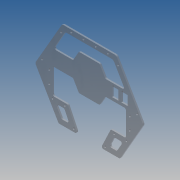
# Autodesk Inventor part: Top Plat
Saved by Autodesk Inventor 2017 (Build 210142000, 142)
## iProperties
Created: 2016-10-14
Part Number: Top Plat
Material: Polycarbonate, Clear
Document SubType Name: Modeling
Designer: James Yelland
Density: 1.2 g/cm^3
Appearance: Polycarbonate - Clear
Author: James Yelland
Autodesk Inventor part; units mm, degrees
ref_plane "YZ Plane" through (0, 0, 0) normal (1, 0, 0) x (0, 1, 0)
ref_plane "XZ Plane" through (0, 0, 0) normal (0, 1, 0) x (-1, 0, 0)
ref_plane "XY Plane" through (0, 0, 0) normal (0, 0, 1) x (1, 0, 0)
sketch "Sketch1" plane through (0, 0, 0) normal (0, 1, 0) x (-1, 0, 0)
  circle A0 centre (-30.6147, -73.9104) radius 1.6
  circle A1 centre (-30.6147, -73.9104) radius 1.6
  line L0 (-103.5566, 2.5) -> (-53.9434, 88.4327)
  line L1 (-49.6132, 90.9327) -> (49.6132, 90.9327)
  line L2 (53.9434, 88.4327) -> (103.5566, 2.5)
  arc A2 (-103.5566, 2.5) -> (-103.5566, -2.5) centre (-99.2265, 0) ccw
  arc A3 (-49.6132, 90.9327) -> (-53.9434, 88.4327) centre (-49.6132, 85.9327) ccw
  arc A4 (53.9434, 88.4327) -> (49.6132, 90.9327) centre (49.6132, 85.9327) ccw
  arc A5 (103.5566, -2.5) -> (103.5566, 2.5) centre (99.2265, 0) ccw
  arc A6 (-43.8396, 80.9325) -> (-48.1698, 78.4325) centre (-43.8396, 75.9325) ccw
  circle A7 centre (-30.6147, -73.9104) radius 1.6
  circle A8 centre (-30.6147, -73.9104) radius 1.6
  arc A9 (48.1698, 78.4325) -> (43.8396, 80.9325) centre (43.8396, 75.9325) ccw
  circle A10 centre (35.5991, 85.9437) radius 1.6
  circle A11 centre (-35.5945, 85.9327) radius 1.6
  circle A12 centre (92.2171, 12.1406) radius 1.6
  circle A13 centre (-92.2171, 12.1406) radius 1.6
  line L3 (-18.2679, -8.3495) -> (18.2679, -8.3495)
  line L4 (-62.8455, -53.0133) -> (-54.5333, -67.4106)
  line L5 (59.1367, 11.2915) -> (33.0718, 11.2915)
  line L6 (59.1367, 11.2915) -> (68.2171, 11.2915)
  line L7 (-62.25, 35.5415) -> (-62.25, 17.0415)
  line L8 (-62.25, 17.0415) -> (-74.75, 17.0415)
  line L9 (-74.75, 17.0415) -> (-74.75, 35.5415)
  line L10 (-74.75, 35.5415) -> (-62.25, 35.5415)
  line L11 (30.4737, 9.7915) -> (20.866, -6.8495)
  line L12 (-30.4737, 9.7915) -> (-20.866, -6.8495)
  arc A14 (33.0718, 11.2915) -> (30.4737, 9.7915) centre (33.0718, 8.2915) ccw
  arc A15 (64.417, 41.2915) -> (67.0151, 45.7915) centre (64.417, 44.2915) ccw
  arc A16 (30.4737, 42.7915) -> (33.0718, 41.2915) centre (33.0718, 44.2915) ccw
  arc A17 (18.2679, -8.3495) -> (20.866, -6.8495) centre (18.2679, -5.3495) ccw
  arc A18 (-20.866, -6.8495) -> (-18.2679, -8.3495) centre (-18.2679, -5.3495) ccw
  arc A19 (-30.4737, 9.7915) -> (-33.0718, 11.2915) centre (-33.0718, 8.2915) ccw
  arc A20 (-33.0718, 41.2915) -> (-30.4737, 42.7915) centre (-33.0718, 44.2915) ccw
  arc A21 (-18.2679, 60.9325) -> (-20.866, 59.4325) centre (-18.2679, 57.9325) ccw
  arc A22 (20.866, 59.4325) -> (18.2679, 60.9325) centre (18.2679, 57.9325) ccw
  arc A23 (-67.0151, 45.7915) -> (-64.417, 41.2915) centre (-64.417, 44.2915) ccw
  line L13 (43.8396, 80.9325) -> (-43.8396, 80.9325)
  line L14 (-48.1698, 78.4325) -> (-67.0151, 45.7915)
  line L15 (-64.417, 41.2915) -> (-33.0718, 41.2915)
  line L16 (-30.4737, 42.7915) -> (-20.866, 59.4325)
  line L17 (-18.2679, 60.9325) -> (18.2679, 60.9325)
  line L18 (20.866, 59.4325) -> (30.4737, 42.7915)
  line L19 (33.0718, 41.2915) -> (64.417, 41.2915)
  line L20 (67.0151, 45.7915) -> (48.1698, 78.4325)
  line L21 (-56.75, 35.5415) -> (-56.75, 17.0415)
  line L22 (-56.75, 17.0415) -> (-44.25, 17.0415)
  line L23 (-44.25, 17.0415) -> (-44.25, 35.5415)
  line L24 (-44.25, 35.5415) -> (-56.75, 35.5415)
  circle A24 centre (-55.4009, 75.9081) radius 1.6
  circle A25 centre (55.3868, 75.9325) radius 1.6
  circle A26 centre (-12, 85.9327) radius 1.6
  circle A27 centre (12, 85.9327) radius 1.6
  circle A28 centre (-78.2171, -22.3594) radius 1.6
  circle A29 centre (-78.2171, 1.6406) radius 1.6
  circle A30 centre (78.2171, -22.3594) radius 1.6
  circle A31 centre (78.2171, 1.6406) radius 1.6
  circle A32 centre (-71.7134, -43.5133) radius 1.6
  circle A33 centre (-47.7134, -43.5133) radius 1.6
  arc A34 (71.2171, 8.2915) -> (68.2171, 11.2915) centre (68.2171, 8.2915) ccw
  line L25 (-33.0718, 11.2915) -> (-68.2171, 11.2915)
  line L26 (-68.2171, -38.5133) -> (-43.8241, -38.5133)
  line L27 (-71.2171, 8.2915) -> (-71.2171, -35.5133)
  arc A35 (-68.2171, 11.2915) -> (-71.2171, 8.2915) centre (-68.2171, 8.2915) ccw
  line L28 (-40.5751, -64.621) -> (-47.4299, -50.2237)
  line L29 (-50.1385, -48.5133) -> (-60.2475, -48.5133)
  arc A36 (-41.1155, -40.2237) -> (-43.8241, -38.5133) centre (-43.8241, -41.5133) ccw
  arc A37 (-47.4299, -50.2237) -> (-50.1385, -48.5133) centre (-50.1385, -51.5133) ccw
  arc A38 (-60.2475, -48.5133) -> (-62.8455, -53.0133) centre (-60.2475, -51.5133) ccw
  arc A39 (-71.2171, -35.5133) -> (-68.2171, -38.5133) centre (-68.2171, -35.5133) ccw
  circle A40 centre (30.6147, -73.9104) radius 1.6
  circle A41 centre (30.6147, -73.9104) radius 1.6
  line L30 (60.303, -77.4174) -> (103.5566, -2.5)
  circle A42 centre (30.6147, -73.9104) radius 1.6
  circle A43 centre (30.6147, -73.9104) radius 1.6
  line L31 (62.8455, -53.0133) -> (54.5294, -67.4174)
  circle A44 centre (47.7134, -43.5133) radius 1.6
  circle A45 centre (71.7134, -43.5133) radius 1.6
  line L32 (68.2171, -38.5133) -> (43.8241, -38.5133)
  line L33 (71.2171, -38.5133) -> (41.9298, -38.5133) construction
  line L34 (71.2171, 8.2915) -> (71.2171, -35.5133)
  line L35 (40.5718, -64.6277) -> (47.4299, -50.2237)
  line L36 (50.1385, -48.5133) -> (60.2475, -48.5133)
  arc A46 (43.8241, -38.5133) -> (41.1155, -40.2237) centre (43.8241, -41.5133) ccw
  arc A47 (50.1385, -48.5133) -> (47.4299, -50.2237) centre (50.1385, -51.5133) ccw
  arc A48 (62.8455, -53.0133) -> (60.2475, -48.5133) centre (60.2475, -51.5133) ccw
  arc A49 (68.2171, -38.5133) -> (71.2171, -35.5133) centre (68.2171, -35.5133) ccw
  line L37 (24.7351, -74.6277) -> (41.1155, -40.2237)
  line L38 (32.3467, -78.9174) -> (57.705, -78.9174)
  line L39 (32.3467, -78.9174) -> (27.4437, -78.9174)
  line L40 (45.0258, -68.9174) -> (43.2805, -68.9174)
  line L41 (45.0258, -68.9174) -> (51.9313, -68.9174)
  arc A50 (24.7351, -74.6277) -> (27.4437, -78.9174) centre (27.4437, -75.9174) ccw
  arc A51 (57.705, -78.9174) -> (60.303, -77.4174) centre (57.705, -75.9174) ccw
  arc A52 (51.9313, -68.9174) -> (54.5294, -67.4174) centre (51.9313, -65.9174) ccw
  arc A53 (40.5718, -64.6277) -> (43.2805, -68.9174) centre (43.2805, -65.9174) ccw
  line L42 (-32.3467, -78.9106) -> (-57.7089, -78.9106)
  line L43 (-45.0278, -68.9106) -> (-51.9352, -68.9106)
  line L44 (-45.0278, -68.9106) -> (-43.2837, -68.9106)
  arc A54 (-43.2837, -68.9106) -> (-40.5751, -64.621) centre (-43.2837, -65.9106) ccw
  arc A55 (-54.5333, -67.4106) -> (-51.9352, -68.9106) centre (-51.9352, -65.9106) ccw
  line L45 (-60.307, -77.4106) -> (-103.5566, -2.5)
  line L46 (-41.1155, -40.2237) -> (-26.1, -71.7609)
  line L47 (-26.1, -71.7609) -> (-24.7383, -74.621)
  line L48 (-27.447, -78.9106) -> (-32.3467, -78.9106)
  arc A56 (-27.447, -78.9106) -> (-24.7383, -74.621) centre (-27.447, -75.9106) ccw
  arc A57 (-60.307, -77.4106) -> (-57.7089, -78.9106) centre (-57.7089, -75.9106) ccw
  point P0 (105, 0)
  point P1 (-105, 0)
  point P2 (-52.5, 90.9327)
  point P3 (52.5, 90.9327)
  point P4 (-46.7264, 80.9325)
  point P5 (46.7264, 80.9325)
  point P6 (-50.7681, -73.9321)
  point P7 (-5, -80.9325)
  point P8 (5, -80.9325)
  point P9 (69.6132, 41.2915)
  point P10 (-69.6132, 41.2915)
  point P11 (0, -8.3495)
  point P12 (0, 90.9327)
  point P13 (-59.7134, -39.5133)
  point P14 (-59.7134, -47.5133)
  point P15 (-70.9879, -38.9104)
  point P16 (-62.905, -52.9104)
  point P17 (-38.1553, -69.7034)
  point P18 (54.8095, -86.9325)
  point P19 (50.7681, -73.9321)
  point P20 (59.7134, -47.5133)
  point P21 (59.7134, -39.5133)
  point P22 (70.9879, -38.9104)
  point P23 (62.905, -52.9104)
  point P24 (38.1553, -69.7034)
  point P25 (24.8278, -74.4329)
  point P26 (22.3467, -78.9174)
  point P27 (53.6633, -68.9174)
  point P28 (-38.5327, -68.9106)
  dimension "d252" = 3.2
  dimension "d254" = 3.2
  dimension "d258" = 3.2
  dimension "d259" = 3.2
  dimension "d263" = 3.2
  dimension "d264" = 3.2
  dimension "d268" = 3.2
  dimension "d269" = 3.2
  dimension "d327" = 3.2
  dimension "d328" = 3.2
  dimension "d336" = 3
  dimension "d339" = 3
  constraints: 98 end point, 69 point on circle, 58 centre point, 26 point on line, 23 tangent, 6 equal radius, 4 coincident, 4 horizontal, 2 midpoint, 1 collinear
  measures "d252" diameter of A26
  measures "d254" diameter of A27
  measures "d258" diameter of A28
  measures "d259" diameter of A29
  measures "d263" diameter of A30
  measures "d264" diameter of A31
  measures "d268" diameter of A32
  measures "d269" diameter of A33
  measures "d327" diameter of A45
  measures "d328" diameter of A44
  measures "d336" radius of A50
  measures "d339" radius of A56
extrude "Extrusion2" add sketch "Sketch1" along normal blind 3
sketch "Sketch2" plane through (0, 3, 0) normal (0, 1, 0) x (1, 0, 0)
  line L0 (-23.051, -6.2915) -> (23.0507, -6.2915) construction
  line L1 (23.0507, -6.2915) -> (23.0507, -46.2915) construction
  line L2 (23.0507, -46.2915) -> (-23.051, -46.2915) construction
  line L3 (-23.051, -46.2915) -> (-23.051, -6.2915) construction
  line L4 (18.2679, 8.3495) -> (-18.2679, 8.3495) projected
  line L5 (-18.2679, -60.9325) -> (18.2679, -60.9325) projected
  line L6 (0, 8.3495) -> (0, -6.2915)
  point P0 (0, 0)
  dimension "d323" = 23.051
  constraints: 2 end point, 1 midpoint, 1 perpendicular, 1 point on line, 2 other
  measures "d323" distance between parallel lines of L3 L6
decal "Decal1"
body "Solid2"
